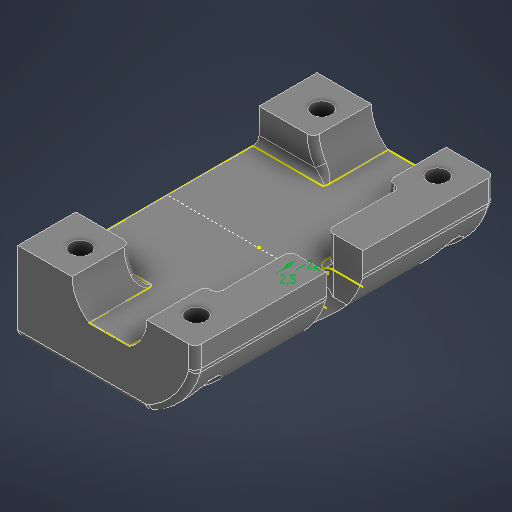
# Autodesk Inventor part: MotorMountBottom
Saved by Autodesk Inventor 2026.2 (Build 302298010, 298A)
## iProperties
Created: 2026-03-29
Part Number: MotorMountBottom
Material: Všeobecné
Document SubType Name: Modeling
Designer: zak
Density: 1 g/cm^3
Appearance: Výchozí
Author: zak
Autodesk Inventor part; units mm, degrees
ref_plane "YZ Plane" through (0, 0, 0) normal (1, 0, 0) x (0, 1, 0)
ref_plane "XZ Plane" through (0, 0, 0) normal (0, 1, 0) x (-1, 0, 0)
ref_plane "XY Plane" through (0, 0, 0) normal (0, 0, 1) x (1, 0, 0)
sketch "Náčrt1" plane through (0, 0, 0) normal (0, 0, 1) x (1, 0, 0)
  circle A0 centre (0, 0) radius 14 construction
  line L0 (-3.3166, 5) -> (3.3166, 5)
  line L1 (-3.3166, -5) -> (3.3166, -5)
  line L2 (-6, 0) -> (6, 0) construction
  line L3 (0, 5) -> (0, -5) construction
  arc A1 (-3.3166, 5) -> (-3.3166, -5) centre (0, 0) ccw
  arc A2 (3.3166, -5) -> (3.3166, 5) centre (0, 0) ccw
  line L4 (3.3541, 5.125) -> (-3.3541, 5.125)
  arc A3 (-3.3541, 5.125) -> (-3.3541, -5.125) centre (0, 0) ccw
  line L5 (-3.3541, -5.125) -> (3.3541, -5.125)
  arc A4 (3.3541, -5.125) -> (3.3541, 5.125) centre (0, 0) ccw
  line L6 (-15, 0) -> (14, 0)
  line L7 (14, 0) -> (14, -13)
  line L8 (14, -13) -> (-15, -13)
  line L9 (-15, -13) -> (-15, 0)
  arc A5 (6.4226, -13) -> (14, -3.7749) centre (0, 0) ccw
  point P0 (-6.125, 0)
  point P1 (6.125, 0)
  dimension "d0" = 28
  dimension "d2" = 10
  dimension "d3" = 6
  dimension "d4" = 0.125
  dimension "d7" = 15
  dimension "d15" = 8
  dimension "d31" = 14
  dimension "d32" = 14.5
  constraints: 20 end point, 12 point on circle, 6 centre point, 4 midpoint, 4 parallel, 3 coincident, 3 horizontal, 2 point on line, 1 collinear, 1 perpendicular, 5 other
  measures "d0" diameter of A0
  measures "d2" distance between parallel lines of L1 L0
  measures "d3" radius of A2
  measures "d4" distance between parallel lines of L0 L4
  measures "d7" distance between parallel lines of L9 L3
  measures "d15" distance between parallel lines of L8 L1
  measures "d31" distance from line of L7 point (0, 0)
  measures "d32" radius of A5
extrude "Vysunutí1" add sketch "Náčrt1" along normal mid plane 49 contours A3 L5 A4 L6 L7 A5 L8 L9
sketch "Náčrt2" plane through (-15, -13, 24.5) normal (0, -1, 0) x (1, 0, 0)
  line L0 (18.3541, -49) -> (18.3541, 0) projected
  line L1 (21.125, 0) -> (18.3541, 0) projected
  line L2 (21.125, -49) -> (21.125, 0) projected
  line L3 (18.3541, -49) -> (21.125, -49) projected
  line L4 (11.6459, 0) -> (11.6459, -49) projected
  line L5 (18.3541, 0) -> (11.6459, 0) projected
  line L6 (18.3541, -49) -> (18.3541, 0) projected
  line L7 (11.6459, -49) -> (18.3541, -49) projected
  line L8 (8.875, -49) -> (8.875, 0) projected
  line L9 (11.6459, 0) -> (8.875, 0) projected
  line L10 (11.6459, 0) -> (11.6459, -49) projected
  line L11 (8.875, -49) -> (11.6459, -49) projected
  line L12 (0, 0) -> (21.4226, 0) projected
  line L13 (0, -49) -> (0, 0) projected
  line L14 (21.4226, -49) -> (0, -49) projected
  circle A0 centre (24.5, -4.75) radius 1.6
  circle A1 centre (5.5, -4.75) radius 1.6
  line L15 (21.4226, -49) -> (21.4226, 0) projected
  point P0 (15, -24.5)
  point P1 (15, 0)
  dimension "d10" = 19
  dimension "d11" = 3.2
  dimension "d12" = 3.2
  dimension "d13" = 4.75
  dimension "d14" = 9.5
  constraints: 2 centre point, 1 horizontal alignment, 1 midpoint
  measures "d10" distance of A1.centre A0.centre
  measures "d11" diameter of A0
  measures "d12" diameter of A1
  measures "d13" distance from line of L12 A0.centre
  measures "d14" horizontal distance of point (15, 0) A0.centre
hole "Díra1" at (-9.5, -13, 19.75) direction (0, 1, 0) diameter 6 depth 2
sketch "Náčrt3" plane through (-9.5, -11, 19.75) normal (0, -1, 0) x (1, 0, 0)
  circle A0 centre (0, 0) radius 3 projected
  point P0 (9.5, -19.75)
  constraints: 1 coincident
hole "Díra3" at (-9.5, -11, 19.75) direction (0, 1, 0) diameter 3.2 end through all countersink diameter 6 countersink angle 90
hole "Díra4" at (9.5, -13, 19.75) direction (0, 1, 0) diameter 6 depth 5.65
sketch "Náčrt4" plane through (9.5, -7.35, 19.75) normal (0, -1, 0) x (1, 0, 0)
  arc A0 (2.9991, 0.0735) -> (2.9991, -0.0735) centre (0, 0) ccw projected
  point P0 (-9.5, -19.75)
  constraints: 1 coincident
hole "Díra5" at (9.5, -7.35, 19.75) direction (0, 1, 0) diameter 3.2 end through all countersink diameter 6 countersink angle 90
mirror "Zrcadlit2" about plane through (0, 0, 0) normal (0, 0, 1) of "Díra1", "Díra3", "Díra4", "Díra5"
sketch "Náčrt5" plane through (6.125, 0, 24.5) normal (0, 1, 0) x (1, 0, 0)
  circle A0 centre (3.375, 44.25) radius 1.6 projected
  circle A1 centre (3.375, 4.75) radius 1.6 projected
  line L0 (0, 49) -> (0, 0) projected
  line L1 (7.875, 0) -> (0, 0) projected
  line L2 (7.875, 49) -> (7.875, 0) projected
  line L3 (0, 49) -> (7.875, 49) projected
  circle A2 centre (-15.625, 44.25) radius 1.6 projected
  circle A3 centre (-15.625, 4.75) radius 1.6 projected
  line L4 (-21.125, 49) -> (-21.125, 0) projected
  line L5 (-12.25, 0) -> (-21.125, 0) projected
  line L6 (-12.25, 49) -> (-12.25, 0) projected
  line L7 (-21.125, 49) -> (-12.25, 49) projected
  line L8 (-12.25, 49) -> (-12.25, 0) projected
  line L9 (-9.4791, 0) -> (-12.25, 0) projected
  line L10 (-9.4791, 0) -> (-9.4791, 49) projected
  line L11 (-12.25, 49) -> (-9.4791, 49) projected
  line L12 (-9.4791, 0) -> (-9.4791, 49) projected
  line L13 (-2.7709, 0) -> (-9.4791, 0) projected
  line L14 (-2.7709, 49) -> (-2.7709, 0) projected
  line L15 (-9.4791, 49) -> (-2.7709, 49) projected
  line L16 (-2.7709, 49) -> (-2.7709, 0) projected
  line L17 (0, 0) -> (-2.7709, 0) projected
  line L18 (0, 49) -> (0, 0) projected
  line L19 (-2.7709, 49) -> (0, 49) projected
  line L20 (-21.125, 39.5) -> (2, 39.5)
  line L21 (2, 39.5) -> (2, 9.5)
  line L22 (2, 9.5) -> (-21.125, 9.5)
  line L23 (-21.125, 9.5) -> (-21.125, 39.5)
  line L24 (-21.125, 24.5) -> (7.875, 24.5) construction
  point P0 (-6.125, 24.5)
  dimension "d54" = 9.5
  dimension "d55" = 2
  constraints: 10 end point, 2 midpoint, 2 parallel, 1 horizontal, 1 perpendicular, 1 point on line, 1 other
  measures "d54" distance between parallel lines of L15 L20
  measures "d55" distance between parallel lines of L0 L21
extrude "Vysunutí2" cut sketch "Náčrt5" against normal up to surface (5.125 mm away) contours L20 L21 L22 L0 | L0 L22 L14 L20 | L14 L22 L10 L20 | L10 L22 L6 L20 | L6 L22 L4 L20
sketch "Náčrt6" plane through (14, -3.7749, 24.5) normal (1, 0, 0) x (0, 0, -1)
  line L0 (49, 3.7749) -> (0, 3.7749) projected
  line L1 (0, 0) -> (0, 3.7749) projected
  line L2 (49, 0) -> (0, 0) projected
  line L3 (49, 3.7749) -> (49, 0) projected
  line L4 (49, -9.2251) -> (0, -9.2251) projected
  line L5 (49, 0) -> (49, -9.2251) projected
  line L6 (49, 0) -> (0, 0) projected
  line L7 (0, -9.2251) -> (0, 0) projected
  circle A0 centre (24.5, -5.2251) radius 1.6
  circle A1 centre (24.5, -5.2251) radius 3
  circle A2 centre (24.5, -5.2251) radius 2.025
  line L8 (24.5, 3.7749) -> (24.5, -9.2251) construction
  dimension "d58" = 3.2
  dimension "d59" = 6
  dimension "d62" = 4.05
  dimension "d88" = 4
  constraints: 4 horizontal alignment, 3 centre point, 2 coincident, 2 end point, 1 midpoint
  measures "d58" diameter of A0
  measures "d59" diameter of A1
  measures "d62" diameter of A2
  measures "d88" distance from line of A1.centre L4
extrude "Vysunutí3" cut sketch "Náčrt6" against normal blind 13 contours A0 | A1 | A2
extrude "Vysunutí4" cut sketch "Náčrt6" against normal through all contours A0 | A2
sketch "Náčrt7" plane through (6.125, 0, 24.5) normal (0, 1, 0) x (1, 0, 0)
  line L0 (0, 39.5) -> (2, 39.5) projected
  line L1 (2, 39.5) -> (2, 9.5) projected
  line L2 (2, 9.5) -> (0, 9.5) projected
  line L3 (0, 9.5) -> (0, 0) projected
  line L4 (7.875, 0) -> (0, 0) projected
  line L5 (7.875, 49) -> (7.875, 0) projected
  line L6 (0, 49) -> (7.875, 49) projected
  line L7 (0, 49) -> (0, 39.5) projected
  circle A0 centre (3.375, 4.75) radius 1.6 projected
  circle A1 centre (3.375, 44.25) radius 1.6 projected
  line L8 (-2.7709, 49) -> (-2.7709, 39.5) projected
  line L9 (-9.4791, 49) -> (-2.7709, 49) projected
  line L10 (-9.4791, 39.5) -> (-9.4791, 49) projected
  line L11 (-21.125, 39.5) -> (-9.4791, 39.5) projected
  line L12 (-21.125, 9.5) -> (-21.125, 39.5) projected
  line L13 (-9.4791, 9.5) -> (-21.125, 9.5) projected
  line L14 (-9.4791, 0) -> (-9.4791, 9.5) projected
  line L15 (-2.7709, 0) -> (-9.4791, 0) projected
  line L16 (-2.7709, 9.5) -> (-2.7709, 0) projected
  line L17 (2, 9.5) -> (-2.7709, 9.5) projected
  line L18 (2, 39.5) -> (2, 9.5) projected
  line L19 (-2.7709, 39.5) -> (2, 39.5) projected
  line L20 (-21.125, 24.5) -> (7.875, 24.5) construction
  line L21 (-7.8693, 27.5) -> (7.875, 27.5)
  line L22 (7.875, 27.5) -> (7.875, 21.5)
  line L23 (7.875, 21.5) -> (-7.8693, 21.5)
  line L24 (-7.8693, 21.5) -> (-7.8693, 27.5)
  line L25 (-7.8693, 27.5) -> (7.875, 21.5) construction
  line L26 (7.875, 27.5) -> (-7.8693, 21.5) construction
  point P0 (-6.125, 24.5)
  point P1 (0.0029, 24.5)
  point P2 (2, 21.5)
  point P3 (7.875, 21.5)
  point P4 (7.875, 27.5)
  point P5 (2, 27.5)
  dimension "d65" = 6
  constraints: 14 end point, 4 midpoint, 2 parallel, 1 collinear, 1 horizontal, 1 perpendicular, 1 point on line
  measures "d65" distance between parallel lines of L23 L21
extrude "Vysunutí5" cut sketch "Náčrt7" against normal blind 9 contours L21 L5 L23 L1
fillet "Zaoblení1" radius 2 3 edges at (14, -3.7749, 13.75) (14, -3.7749, -13.75) (6.4226, -13, 0)
fillet "Zaoblení2" radius 1 10 edges at (13.9799, -3.7828, 24.5) (14, -1.75, 24.5) (6.4271, -12.9391, 24.5) (-4.5314, -13, 24.5) (11.2764, -9.1156, 24.5) (6.4271, -12.9391, -24.5) (-4.5314, -13, -24.5) (13.9799, -3.7828, -24.5) (14, -1.75, -24.5) (11.2764, -9.1156, -24.5)
fillet "Zaoblení3" radius 1 4 edges at (8.125, -2.5625, -3) (8.125, -7.0625, -3) (8.125, -2.5625, 3) (8.125, -7.0625, 3)
fillet "Zaoblení4" radius 1 14 edges at (-9.1771, -5.125, -15) (-5.3879, -2.9131, -15) (-5.3879, -2.9131, 15) (-9.1771, -5.125, 15) (5.3879, -2.9131, 15) (5.7396, -5.125, 15) (8.125, -2.5625, 15) (8.4179, -5.125, 3.2929) (8.125, -5.125, 9.5) (5.7396, -5.125, -15) (8.125, -2.5625, -15) (8.4179, -5.125, -3.2929) (8.125, -5.125, -9.5) (5.3879, -2.9131, -15)
sketch "Náčrt8" plane through (-15, 0, 15) normal (-1, 0, 0) x (0, 0, 1)
  circle A0 centre (-15, -9) radius 2.025 projected
  arc A1 (-39.5, -12) -> (-38.5, -13) centre (-38.5, -12) ccw projected
  line L0 (-38.5, -13) -> (8.5, -13) projected
  arc A2 (8.5, -13) -> (9.5, -12) centre (8.5, -12) ccw projected
  line L1 (9.5, 0) -> (9.5, -12) projected
  line L2 (0, 0) -> (9.5, 0) projected
  line L3 (0, 0) -> (0, -4.125) projected
  arc A3 (-1, -5.125) -> (0, -4.125) centre (-1, -4.125) ccw projected
  line L4 (-1, -5.125) -> (-29, -5.125) projected
  arc A4 (-30, -4.125) -> (-29, -5.125) centre (-29, -4.125) ccw projected
  line L5 (-30, -4.125) -> (-30, 0) projected
  line L6 (-39.5, 0) -> (-30, 0) projected
  line L7 (-39.5, -12) -> (-39.5, 0) projected
  circle A5 centre (-15, -9) radius 2.025 projected
  line L8 (-1, -5.125) -> (-29, -5.125) projected
  arc A6 (-27.4933, -8) -> (-26.8779, -13) centre (-15, -9) ccw
  arc A7 (-3.1221, -13) -> (-2.5067, -8) centre (-15, -9) ccw
  arc A8 (-30, -8) -> (-29.4914, -13) centre (-15, -9) ccw
  arc A9 (-0.5086, -13) -> (0, -8) centre (-15, -9) ccw
  line L9 (-15, -5.125) -> (-15, -13) construction
  line L10 (-30, -8) -> (-27.4933, -8)
  line L11 (-2.5067, -8) -> (0, -8)
  point P0 (-15, 0)
  dimension "d78" = 1
  dimension "d81" = 2.5
  constraints: 8 point on circle, 6 end point, 4 centre point, 4 point on line, 2 coincident, 2 midpoint, 2 parallel, 1 vertical alignment, 3 other
  measures "d78" distance from line of L10 A0.centre
  measures "d81" radial gap between concentric circles of A8 A6
extrude "Vysunutí6" cut sketch "Náčrt8" against normal blind 4 contours A8 L10 A6 L0 | A7 L11 A9 L0
offset faces "Velikost1" outward -0.125 faces at (-13.6667, -8.5604, -15.0269) (-13.6667, -12.462, -12.0457) (-12.3333, -8.5604, 15.0269) (-12.3333, -10.8105, 12.4018)
fillet "Zaoblení5" radius 0.5 2 edges at (-13, -13, -11.7459) (-13, -13, 11.7459)
fillet "Zaoblení5" radius 0.25 2 edges at (-13, -13, -14.621) (-13, -13, 14.621)
fillet "Zaoblení5" radius 0.75 4 edges at (-13, -8, 12.3679) (-13, -8, 15.1253) (-13, -8, -12.3679) (-13, -8, -15.1253)
sketch "Náčrt9" plane through (-3.3541, -5.125, -24.5) normal (0, 1, 0) x (1, 0, 0)
  arc A0 (10.4791, -20.5) -> (11.5109, -22.25) centre (12.4791, -20.5) ccw projected
  line L0 (10.4791, -10.5) -> (10.4791, -20.5) projected
  line L1 (6.9942, -10.5) -> (10.4791, -10.5) projected
  line L2 (6.7082, 0) -> (6.7082, -9.7085) projected
  line L3 (0, 0) -> (6.7082, 0) projected
  line L4 (0, -9.7085) -> (0, 0) projected
  line L5 (-11.6459, -10.5) -> (-0.286, -10.5) projected
  line L6 (-11.6459, -38.5) -> (-11.6459, -10.5) projected
  line L7 (-0.286, -38.5) -> (-11.6459, -38.5) projected
  line L8 (0, -49) -> (0, -39.2915) projected
  line L9 (6.7082, -49) -> (0, -49) projected
  line L10 (6.7082, -39.2915) -> (6.7082, -49) projected
  line L11 (10.4791, -38.5) -> (6.9942, -38.5) projected
  line L12 (10.4791, -28.5) -> (10.4791, -38.5) projected
  arc A1 (11.5109, -26.75) -> (10.4791, -28.5) centre (12.4791, -28.5) ccw projected
  arc A2 (11.4791, -26.5) -> (11.5109, -26.75) centre (12.4791, -26.5) ccw projected
  line L13 (11.4791, -22.5) -> (11.4791, -26.5) projected
  arc A3 (11.5109, -22.25) -> (11.4791, -22.5) centre (12.4791, -22.5) ccw projected
  line L14 (12.4791, -21.5) -> (17.3541, -21.5) projected
  line L15 (17.3541, -27.5) -> (12.4791, -27.5) projected
  arc A4 (12.4791, -27.5) -> (11.4791, -28.5) centre (12.4791, -28.5) ccw projected
  arc A5 (11.4791, -20.5) -> (12.4791, -21.5) centre (12.4791, -20.5) ccw projected
  line L16 (11.4791, -24.5) -> (-11.6459, -24.5) construction
  circle A6 centre (8.2291, -24.5) radius 1.25
  point P0 (3.3541, -24.5)
  dimension "d86" = 2.5
  dimension "d87" = 2
  constraints: 2 end point, 2 midpoint, 1 centre point, 1 point on line, 6 other
  measures "d86" diameter of A6
  measures "d87" distance edge to line of A6 L13
equation "\"d12\" = d11"
